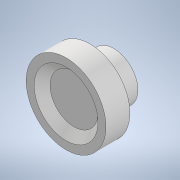
# Autodesk Inventor part: encoder_ma_holder
Saved by Autodesk Inventor 2020 (Build 240168000, 168)
## iProperties
Created: 2019-10-19
Part Number: encoder_ma_holder
Material: Generic
Document SubType Name: Modeling
Designer: psrob
Density: 1 g/cm^3
Appearance: Default
Author: psrob
Autodesk Inventor part; units mm, degrees
ref_plane "YZ Plane" through (0, 0, 0) normal (1, 0, 0) x (0, 1, 0)
ref_plane "XZ Plane" through (0, 0, 0) normal (0, 1, 0) x (-1, 0, 0)
ref_plane "XY Plane" through (0, 0, 0) normal (0, 0, 1) x (1, 0, 0)
sketch "Sketch1" plane through (0, 0, 0) normal (0, 0, 1) x (1, 0, 0)
  circle A0 centre (0, 0) radius 3 projected
  circle A1 centre (0, 0) radius 3
  point P0 (0, 0)
  dimension "d0" = 6
  constraints: 1 centre point, 1 coincident
  measures "d0" diameter of A1
extrude "Extrusion1" add sketch "Sketch1" against normal blind 3
sketch "Sketch2" plane through (0, 0, 0) normal (0, 0, 1) x (1, 0, 0)
  circle A0 centre (0, 0) radius 3 projected
  circle A1 centre (0, 0) radius 11 projected
  circle A2 centre (0, 0) radius 3 projected
  circle A3 centre (8, 0) radius 1.5 projected
  circle A4 centre (0, 8) radius 1.5 projected
  circle A5 centre (-8, 0) radius 1.5 projected
  circle A6 centre (0, -8) radius 1.5 projected
  circle A7 centre (0, 0) radius 5
  point P0 (0, 0)
  dimension "d3" = 10
  constraints: 1 centre point, 1 coincident
  measures "d3" diameter of A7
extrude "Extrusion2" add sketch "Sketch2" along normal blind 2 contours A0 | A7
sketch "Sketch3" plane through (0, 0, 2) normal (0, 0, 1) x (1, 0, 0)
  circle A0 centre (0, 0) radius 5 projected
  circle A1 centre (0, 0) radius 3 projected
  circle A2 centre (0, 0) radius 3
  point P0 (0, 0)
  dimension "d6" = 6
  constraints: 1 centre point, 1 coincident
  measures "d6" diameter of A2
extrude "Extrusion3" add sketch "Sketch3" along normal blind 1
chamfer "Chamfer1" distance 1 angle 45 1 edges at (-3, 0, 3)
thicken "Thicken1" operation add thickness 0.05 both sides no extend neighbours yes toward (-0.9967573, 0.0804666, 0) faces at (2.9903, -0.2414, -2)
chamfer "Chamfer2" distance 0.5 angle 45 1 edges at (-2.95, 0, -3)
body "Solid1"
